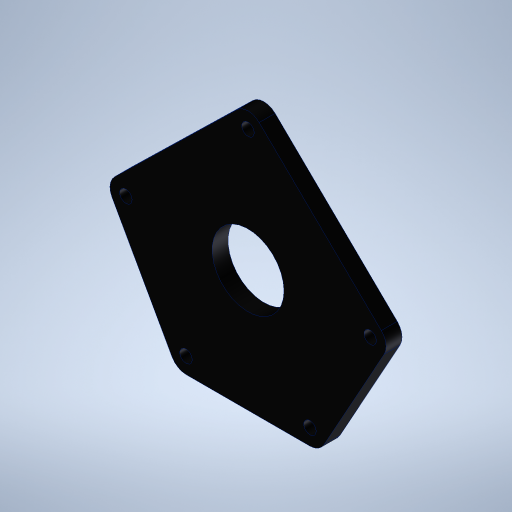
# Autodesk Inventor part: TopPlate_Gearboxes_2_Exercise_2
Saved by Autodesk Inventor 2024 (Build 280153000, 153)
## iProperties
Created: 2024-11-16
Part Number: TopPlate_Gearboxes_2_Exercise_2
Material: Aluminum 6061
Document SubType Name: Modeling
Designer: Danielle
Density: 2.7 g/cm^3
Appearance: Aluminum - Flat
Author: Danielle
Autodesk Inventor part; units mm, degrees
ref_plane "YZ Plane" through (0, 0, 0) normal (1, 0, 0) x (0, 1, 0)
ref_plane "XZ Plane" through (0, 0, 0) normal (0, 1, 0) x (-1, 0, 0)
ref_plane "XY Plane" through (0, 0, 0) normal (0, 0, 1) x (1, 0, 0)
sketch "Sketch1" plane through (0, 0, 0) normal (0, 0, 1) x (1, 0, 0)
  circle A0 centre (0, 0) radius 38.1 construction
  circle A1 centre (0, 0) radius 40.64 construction
  circle A2 centre (0, 0) radius 14.2875
  circle A3 centre (-31.9157, 32.7369) radius 30.0609 construction
  circle A4 centre (-31.9157, 32.7369) radius 25.4 construction
  circle A5 centre (-31.9157, 32.7369) radius 7.62 construction
  line L0 (-52.4066, 17.305) -> (0, 0) construction
  line L1 (0, 0) -> (-17.9111, 52.2025) construction
  circle A6 centre (-48.5745, 1.2342) radius 2.4892
  circle A7 centre (-48.5745, 1.2342) radius 6.35 construction
  circle A8 centre (-48.5745, 1.2342) radius 3.9751 construction
  line L2 (-46.7163, 4.7482) -> (-45.9682, 6.1628) construction
  line L3 (-42.2266, 1.0729) -> (-40.6269, 1.0322) construction
  circle A9 centre (0, 48.5902) radius 6.35 construction
  circle A10 centre (0, 48.5902) radius 3.9751 construction
  circle A11 centre (0, 48.5902) radius 2.4892
  line L4 (0, 42.2402) -> (0, 40.64) construction
  line L5 (-3.5601, 46.8218) -> (-4.9932, 46.1099) construction
  circle A12 centre (-24.6505, -41.8731) radius 6.35 construction
  circle A13 centre (-24.6505, -41.8731) radius 2.4892
  line L6 (-21.4291, -36.4009) -> (-20.6173, -35.022)
  line L7 (0, 48.5902) -> (0, 0) construction
  circle A14 centre (31.9157, 32.7369) radius 30.0609 construction
  circle A15 centre (31.9157, 32.7369) radius 25.4 construction
  circle A16 centre (48.5745, 1.2342) radius 2.4892
  circle A17 centre (48.5745, 1.2342) radius 6.35 construction
  circle A18 centre (48.5745, 1.2342) radius 3.9751 construction
  circle A19 centre (0, 48.5902) radius 2.4892 construction
  circle A20 centre (24.6505, -41.8731) radius 6.35 construction
  circle A21 centre (24.6505, -41.8731) radius 2.4892
  circle A22 centre (31.9157, 32.7369) radius 7.62 construction
  line L8 (-48.5745, 1.2342) -> (-24.6505, -41.8731) construction
  line L9 (24.6505, -41.8731) -> (-24.6505, -41.8731) construction
  circle A23 centre (-31.9157, 32.7369) radius 10.3188
  circle A24 centre (31.9157, 32.7369) radius 10.3188
  line L10 (-54.1268, -1.8472) -> (-30.2028, -44.9545)
  line L11 (-24.6505, -48.2231) -> (24.6505, -48.2231)
  line L12 (30.2028, -44.9545) -> (54.1268, -1.8472)
  arc A25 (-30.2028, -44.9545) -> (-24.6505, -48.2231) centre (-24.6505, -41.8731) ccw
  arc A26 (-53.0073, 5.781) -> (-54.1268, -1.8472) centre (-48.5745, 1.2342) ccw
  arc A27 (54.1268, -1.8472) -> (53.0073, 5.781) centre (48.5745, 1.2342) ccw
  arc A28 (24.6505, -48.2231) -> (30.2028, -44.9545) centre (24.6505, -41.8731) ccw
  line L13 (-4.4327, 53.137) -> (-53.0073, 5.781)
  line L14 (4.4327, 53.137) -> (53.0073, 5.781)
  arc A29 (4.4327, 53.137) -> (-4.4327, 53.137) centre (0, 48.5902) ccw
  arc A30 (4.4327, 53.137) -> (-4.4327, 53.137) centre (0, 48.5902) ccw
  dimension "d15" = 7.9502
  dimension "d0" = 76.2
  dimension "d1" = 2.54
  dimension "d2" = 28.575
  dimension "d3" = 60.1218
  dimension "d4" = 50.8
  dimension "d5" = 15.24
  dimension "d12" = 12.7
  dimension "d14" = 4.9784
  dimension "d16" = 1.6002
  dimension "d17" = 15.24
  dimension "d18" = 20.6375
  dimension "d19" = 20.6375
  constraints: 30 end point, 28 centre point, 28 point on circle, 15 coincident, 14 tangent, 10 point on line, 8 symmetric about line, 6 equal length, 4 equal radius, 3 concentric, 2 horizontal, 2 vertical, 19 other
  measures "d0" diameter of A0
  measures "d1" radial gap between concentric circles of A1 A0
  measures "d2" diameter of A2
  measures "d3" diameter of A3
  measures "d4" diameter of A4
  measures "d5" diameter of A5
  measures "d12" diameter of A7
  measures "d14" diameter of A6
  measures "d16" distance of L2.start L2.end
  measures "d17" diameter of A22
  measures "d18" diameter of A23
  measures "d19" diameter of A24
extrude "Extrusion2" add sketch "Sketch1" along normal blind 6.35 contours A23 L13 | A23 L13 A29 L14 A24 A27 L12 A28 L11 A25 L10 A26 | L14 A24 picked at (-26.2947, 29.0376) picked at (27.7057, 27.8118)
body "Solid2"
